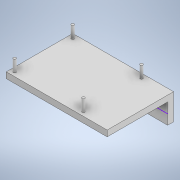
# Autodesk Inventor part: 라즈베리파이 케이스
Saved by Autodesk Inventor 2022 (Build 260153000, 153)
## iProperties
Created: 2024-01-09
Part Number: 라즈베리파이 케이스
Material: 일반
Document SubType Name: Modeling
Designer: slskz
Density: 1 g/cm^3
Appearance: 기본값
Author: slskz
Autodesk Inventor part; units mm, degrees
ref_plane "YZ Plane" through (0, 0, 0) normal (1, 0, 0) x (0, 1, 0)
ref_plane "XZ Plane" through (0, 0, 0) normal (0, 1, 0) x (-1, 0, 0)
ref_plane "XY Plane" through (0, 0, 0) normal (0, 0, 1) x (1, 0, 0)
sketch "스케치1" plane through (0, 0, 0) normal (0, 1, 0) x (-1, 0, 0)
  point P0 (0, 0)
sketch "스케치2" plane through (0, 0, 0) normal (0, 1, 0) x (-1, 0, 0)
  line L0 (-42.5, 28) -> (42.5, 28)
  line L1 (42.5, 28) -> (42.5, -28)
  line L2 (42.5, -28) -> (-42.5, -28)
  line L3 (-42.5, -28) -> (-42.5, 28)
  line L4 (-42.5, 28) -> (42.5, -28) construction
  line L5 (42.5, 28) -> (-42.5, -28) construction
  point P0 (0, 0)
  dimension "d0" = 85
  dimension "d1" = 56
  constraints: 12 end point, 2 midpoint, 2 parallel, 1 horizontal, 1 perpendicular
  measures "d0" distance of L1.end L2.end
  measures "d1" distance of L0.end L1.end
extrude "돌출1" add sketch "스케치2" along normal blind 5
sketch "스케치3" plane through (0, 5, 0) normal (0, 1, 0) x (1, 0, 0)
  circle A0 centre (-39, -24.5) radius 1.15
  circle A1 centre (-39, 24.5) radius 1.15
  circle A2 centre (19, 24.5) radius 1.15
  circle A3 centre (19, -24.5) radius 1.15
  line L0 (-42.5, 28) -> (-42.5, -28) projected
  line L1 (-42.5, -28) -> (42.5, -28) projected
  line L2 (42.5, 28) -> (-42.5, 28) projected
  point P0 (0, 0)
  dimension "d4" = 2.3
  dimension "d5" = 2.3
  dimension "d6" = 2.3
  dimension "d7" = 2.3
  dimension "d8" = 3.5
  dimension "d9" = 3.5
  dimension "d10" = 3.5
  dimension "d11" = 3.5
  dimension "d12" = 58
  dimension "d13" = 58
  dimension "d14" = 3.5
  dimension "d15" = 3.5
  constraints: 4 centre point
  measures "d4" diameter of A0
  measures "d5" diameter of A1
  measures "d6" diameter of A2
  measures "d7" diameter of A3
  measures "d8" distance from line of A0.centre L0
  measures "d9" distance from line of L1 A0.centre
  measures "d10" distance from line of A1.centre L0
  measures "d11" distance from line of L2 A1.centre
  measures "d12" distance of A2.centre A1.centre
  measures "d13" distance of A3.centre A0.centre
  measures "d14" distance from line of L2 A2.centre
  measures "d15" distance from line of L1 A3.centre
extrude "돌출2" add sketch "스케치3" along normal blind 10
sketch "스케치4" plane through (0, 0, 0) normal (0, 0, 1) x (1, 0, 0)
  point P0 (0, 0)
sketch "스케치5" plane through (0, 0, 0) normal (0, -1, 0) x (1, 0, 0)
  line L0 (42.5, 28) -> (42.5, -28) projected
  line L1 (-42.5, -28) -> (-42.5, 28) projected
  line L2 (42.5, -23) -> (-42.5, -23)
  line L3 (-42.5, -23) -> (-42.5, -28)
  line L4 (-42.5, -28) -> (42.5, -28)
  line L5 (42.5, -28) -> (42.5, -23)
  point P0 (0, 0)
  dimension "d20" = 5
  constraints: 8 end point, 2 parallel, 1 horizontal, 1 perpendicular, 1 point on line
  measures "d20" distance between parallel lines of L2 L4
extrude "돌출3" add sketch "스케치5" along normal blind 17
sketch "스케치6" plane through (-42.5, 0, -23) normal (0, 0, 1) x (1, 0, 0)
  line L0 (0, -17) -> (0, 5) projected
  line L1 (0, -8.6067) -> (85.0901, -8.6067)
  point P0 (42.5, 0)
  constraints: 2 end point, 1 horizontal, 1 point on line
sketch "스케치7" plane through (-42.5, 0, -23) normal (0, 0, 1) x (1, 0, 0)
  point P0 (42.5, 0)
  point P1 (11.4795, -8.6132)
  point P2 (72.2803, -8.5393)
hole "구멍1" at (-31.0205, -8.6132, -23) at (29.7803, -8.5393, -23) direction (0, 0, -1) diameter 5.5 end through all clearance for "Hex Head Cap Screw" size "M5" standard "Ansi Metric M Profile"
